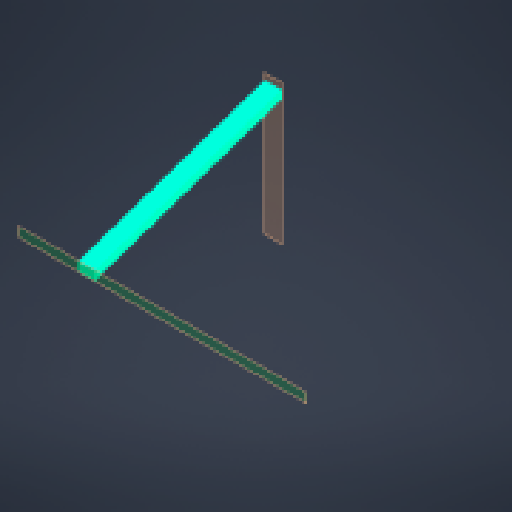
# Autodesk Inventor part: UpperEarDiagonalv2
Saved by Autodesk Inventor 2027 (Build 310192000, 192)
## iProperties
Created: 2026-08-07
Part Number: UpperEarDiagonalv2
Material: Generic
Document SubType Name: Modeling
Designer: lucas
Density: 1 g/cm^3
Appearance: Default
Author: lucas
Autodesk Inventor part; units mm, degrees
ref_plane "YZ Plane" through (0, 0, 0) normal (1, 0, 0) x (0, 1, 0)
ref_plane "XZ Plane" through (0, 0, 0) normal (0, 1, 0) x (-1, 0, 0)
ref_plane "XY Plane" through (0, 0, 0) normal (0, 0, 1) x (1, 0, 0)
ref_plane "Work Plane1" through (0, 0, 0) normal (0, 0, 1) x (1, 0, 0)
sketch "Sketch1" plane through (0, 0, 0) normal (0, 0, 1) x (1, 0, 0)
  line L0 (0, 762) -> (101.6, 762)
  line L1 (101.6, 762) -> (101.6, 711.2)
  line L2 (101.6, 711.2) -> (0, 711.2)
  line L3 (0, 711.2) -> (0, 762)
  point P0 (0, 0)
  dimension "d0" = 101.6
  dimension "d1" = 50.8
  constraints: 8 end point, 2 parallel, 1 horizontal, 1 perpendicular, 1 other
  measures "d0" distance of L1.end L2.end
  measures "d1" distance of L0.end L1.end
ref_plane "Work Plane2" through (-279.4, 379.7477, 1118.6515) normal (0, -0.0012, -1) x (1, 0, 0)
sketch "Sketch2" plane through (-279.4, 379.7477, 1118.6515) normal (0, -0.0012, -1) x (1, 0, 0)
  line L0 (1574.8, 0) -> (0, 0) projected
  line L1 (381, 378.3558) -> (381, -383.6437) projected
  line L2 (381, 0) -> (279.4, 0)
  line L3 (279.4, 0) -> (279.4, 50.8)
  line L4 (279.4, 50.8) -> (381, 50.8)
  line L5 (381, 50.8) -> (381, 0)
  point P0 (279.4, 378.4162)
  dimension "d2" = 101.6
  dimension "d3" = 50.8
  constraints: 8 end point, 2 parallel, 2 point on line, 1 horizontal, 1 perpendicular
  measures "d2" distance of L3.end L4.end
  measures "d3" distance of L2.end L3.end
loft "Loft1" add profiles "Sketch2", "Sketch1"
body "Solid1"
